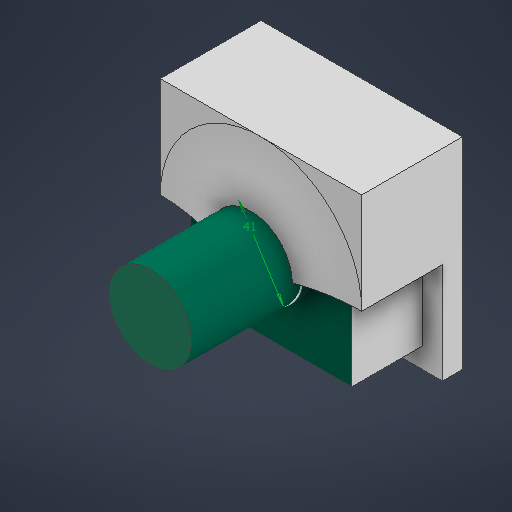
# Autodesk Inventor part: soporte
Saved by Autodesk Inventor 2026.1 (Build 301233020, 233B)
## iProperties
Created: 2026-01-11
Part Number: soporte
Material: Generic
Document SubType Name: Modeling
Designer: Marcelo
Density: 1 g/cm^3
Appearance: Default
Author: Marcelo
Autodesk Inventor part; units mm, degrees
ref_plane "YZ Plane" through (0, 0, 0) normal (1, 0, 0) x (0, 1, 0)
ref_plane "XZ Plane" through (0, 0, 0) normal (0, 1, 0) x (-1, 0, 0)
ref_plane "XY Plane" through (0, 0, 0) normal (0, 0, 1) x (1, 0, 0)
sketch "Sketch1" plane through (0, 0, 0) normal (0, 0, 1) x (1, 0, 0)
  circle A0 centre (0, 0) radius 30
  line L0 (50, -50) -> (-50, -50)
  line L1 (-50, -50) -> (-50, 50)
  line L2 (-50, 50) -> (50, 50)
  line L3 (50, 50) -> (50, -50)
  line L4 (50, -50) -> (-50, 50) construction
  line L5 (-50, -50) -> (50, 50) construction
  dimension "d2" = 60
  dimension "d30" = 100
  dimension "d31" = 100
  constraints: 12 end point, 2 midpoint, 2 parallel, 1 centre point, 1 coincident, 1 horizontal, 1 perpendicular
  measures "d2" diameter of A0
  measures "d30" distance of L1.end L2.end
  measures "d31" distance of L0.end L1.end
extrude "Extrusion1" add sketch "Sketch1" along normal blind 10 contours A0 | L0 L1 L2 L3
sketch "Sketch2" plane through (0, 0, 0) normal (0, 0, -1) x (-1, 0, 0)
  circle A0 centre (0, 0) radius 25 construction
  line L0 (0, 0) -> (-12.5, 21.6506) construction
  line L1 (0, 0) -> (25, 0) construction
  line L2 (0, 0) -> (-25, 0) construction
  line L3 (0, 0) -> (12.5, -21.6506) construction
  line L4 (0, 0) -> (12.5, 21.6506) construction
  line L5 (0, 0) -> (-12.5, -21.6506) construction
  circle A1 centre (12.5, 21.6506) radius 2.5
  circle A2 centre (-12.5, 21.6506) radius 2.5
  circle A3 centre (-25, 0) radius 2.5
  circle A4 centre (-12.5, -21.6506) radius 2.5
  circle A5 centre (12.5, -21.6506) radius 2.5
  circle A6 centre (25, 0) radius 2.5
  dimension "d3" = 50
  dimension "d4" = 60
  dimension "d5" = 60
  dimension "d6" = 60
  dimension "d7" = 60
  dimension "d8" = 60
  dimension "d9" = 5
  dimension "d10" = 5
  dimension "d11" = 5
  dimension "d12" = 5
  dimension "d13" = 5
  dimension "d14" = 5
  constraints: 12 end point, 7 centre point, 6 coincident, 6 point on circle, 1 horizontal
  measures "d3" diameter of A0
  measures "d4" angle of L4 L1
  measures "d5" angle of L3 L1
  measures "d6" angle of L5 L3
  measures "d7" angle of L5 L2
  measures "d8" angle of L0 L2
  measures "d9" diameter of A1
  measures "d10" diameter of A2
  measures "d11" diameter of A3
  measures "d12" diameter of A4
  measures "d13" diameter of A5
  measures "d14" diameter of A6
extrude "Extrusion2" cut sketch "Sketch2" against normal through all
sketch "Sketch8" plane through (0, 0, 0) normal (0, 0, -1) x (-1, 0, 0)
  circle A0 centre (0, 0) radius 30
  circle A1 centre (-12.5, 21.6506) radius 2.5 projected
  circle A2 centre (-25, 0) radius 2.5 projected
  circle A3 centre (-12.5, -21.6506) radius 2.5 projected
  circle A4 centre (12.5, -21.6506) radius 2.5 projected
  circle A5 centre (25, 0) radius 2.5 projected
  circle A6 centre (12.5, 21.6506) radius 2.5 projected
  dimension "d34" = 60
  constraints: 1 centre point, 1 coincident
  measures "d34" diameter of A0
extrude "Extrusion5" add sketch "Sketch8" against normal blind 11
sketch "Sketch9" plane through (0, 0, 10) normal (0, 0, 1) x (1, 0, 0)
  circle A0 centre (0, 0) radius 30 projected
  line L0 (50, 50) -> (-50, 50) projected
  line L1 (-50, 50) -> (-50, -50) projected
  line L2 (-50, -50) -> (50, -50) projected
  line L3 (50, -50) -> (50, 50) projected
  line L4 (-45, -45) -> (-45, 45)
  line L5 (-45, 45) -> (45, 45)
  line L6 (45, 45) -> (45, -45)
  line L7 (45, -45) -> (-45, -45)
  dimension "d37" = 5
  constraints: 8 end point, 3 other
  measures "d37" distance between parallel lines of L1 L4
extrude "Extrusion6" add sketch "Sketch9" along normal blind 40 contours L3 L2 L1 L0
sketch "Sketch10" plane through (0, 0, 50) normal (0, 0, 1) x (1, 0, 0)
  circle A0 centre (0, 0) radius 20.5
  dimension "d40" = 41
  constraints: 1 centre point, 1 coincident
  measures "d40" diameter of A0
sketch "Sketch11" plane through (0, 0, 0) normal (0, 1, 0) x (-1, 0, 0)
  line L0 (45, 50) -> (-45, 50) projected
  line L1 (0, 50) -> (0, 55)
  line L2 (-50, 50) -> (50, 50) projected
  line L3 (-20.5, 55) -> (20.5, 55)
  arc A0 (20.5, 55) -> (50, 50) centre (50, 139.525) ccw
  arc A1 (-50, 50) -> (-20.5, 55) centre (-50, 139.525) ccw
  line L4 (20.5, 55) -> (20.5, 50)
  line L5 (20.5, 50) -> (20.5, 45)
  line L6 (20.5, 45) -> (50, 45)
  line L7 (50, 45) -> (50, 50)
  point P0 (0, 0)
  dimension "d41" = 5
  dimension "d42" = 41
  dimension "d43" = 5
  constraints: 12 end point, 4 perpendicular, 4 point on circle, 2 centre point, 2 midpoint, 2 tangent, 1 horizontal, 1 point on line, 1 vertical
  measures "d41" distance of L1.start L1.end
  measures "d42" distance of L3.start L3.end
  measures "d43" distance of L4.end L5.end
revolve "Revolution2" add sketch "Sketch11" angle 360 about axis through (0, 0, 50) along (0, 0, 1) contours L2 L7 L6 L5 L0 | L0 L4 A0 L2
sketch "Sketch12" plane through (0, 0, 50) normal (0, 0, 1) x (1, 0, 0)
  arc A0 (-21.7945, 45) -> (-45, 21.7945) centre (0, 0) ccw projected
  line L0 (-45, -45) -> (45, -45) projected
  line L1 (45, -45) -> (45, 45) projected
  line L2 (45, 45) -> (-45, 45) projected
  line L3 (-45, 45) -> (-45, -45) projected
  circle A1 centre (0, 0) radius 30 projected
  arc A2 (45, 21.7945) -> (21.7945, 45) centre (0, 0) ccw projected
  arc A3 (21.7945, -45) -> (45, -21.7945) centre (0, 0) ccw projected
  arc A4 (-45, -21.7945) -> (-21.7945, -45) centre (0, 0) ccw projected
  point P0 (-45, 21.7945)
  point P1 (-21.7945, 45)
extrude "Extrusion7" add sketch "Sketch12" against normal blind 5 contours A0 L3 L2 | L2 L1 A2 | A4 L0 L3 | L1 L0 A3
sketch "Sketch13" plane through (0, 0, 0) normal (0, 1, 0) x (-1, 0, 0)
  line L0 (45, 10) -> (45, 45) projected
  line L1 (45, 10) -> (50, 10)
  line L2 (50, 0) -> (50, 50) projected
  line L3 (50, 10) -> (50, 79.5964)
  line L4 (50, 79.5964) -> (-50, 79.5964)
  line L5 (-45, 10) -> (-45, 45) projected
  line L6 (-45, 10) -> (-50, 10)
  line L7 (-50, 0) -> (-50, 50) projected
  line L8 (-50, 10) -> (-50, 79.5964)
  line L9 (-45, 10) -> (45, 10) projected
  line L10 (30, 11) -> (-30, 11) projected
  line L11 (30, 10) -> (30, 11) projected
  line L12 (-30, 10) -> (-30, 11) projected
  point P0 (0, 0)
  dimension "d47" = 100
  constraints: 10 end point, 2 horizontal, 2 point on line, 1 collinear, 1 perpendicular
  measures "d47" distance of L3.end L4.end
extrude "Extrusion8" cut sketch "Sketch13" against normal through all contours L9 L11 L10 L12 L6 L7 L8 L4 L3 L2 L1
sketch "Sketch14" plane through (-50, -50, 0) normal (0, -1, 0) x (1, 0, 0)
  line L0 (80, 11) -> (20, 11) projected
  line L1 (100, 10) -> (80, 10) projected
  line L2 (20, 11) -> (80, 11)
  line L3 (80, 11) -> (80, 10)
  line L4 (80, 10) -> (20, 10)
  line L5 (20, 10) -> (20, 11)
  point P0 (50, 0)
  constraints: 8 end point, 2 parallel, 1 horizontal, 1 perpendicular
extrude "Extrusion9" cut sketch "Sketch14" against normal blind 10
sketch "Sketch15" plane through (0, 0, 10) normal (0, 0, 1) x (1, 0, 0)
  line L0 (40, -40) -> (-40, -40)
  line L1 (-40, -40) -> (-40, 40)
  line L2 (-40, 40) -> (40, 40)
  line L3 (40, 40) -> (40, -40)
  line L4 (40, -40) -> (-40, 40) construction
  line L5 (-40, -40) -> (40, 40) construction
  point P0 (0, 0)
  dimension "d52" = 80
  dimension "d53" = 80
  constraints: 12 end point, 2 midpoint, 2 parallel, 1 horizontal, 1 perpendicular
  measures "d52" distance of L1.end L2.end
  measures "d53" distance of L0.end L1.end
extrude "Extrusion10" add sketch "Sketch15" along normal blind 35
sketch "Sketch16" plane through (0, 0, 45) normal (0, 0, 1) x (1, 0, 0)
  arc A0 (20.5, 0) -> (-20.5, 0) centre (0, 0) ccw projected
  circle A1 centre (0, 0) radius 20.5
  point P0 (-20.5, 0)
  constraints: 1 centre point, 1 coincident
extrude "Extrusion11" add sketch "Sketch16" along normal blind 60
body "Solid1"
